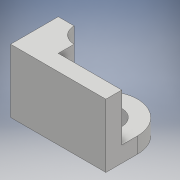
# Autodesk Inventor part: 7
Saved by Autodesk Inventor 2017 (Build 210142000, 142)
## iProperties
Part Number: 7
Material: 一般
Document SubType Name: Modeling
Designer: Brian
Density: 1 g/cm^3
Appearance: 預設
Author: Brian
Autodesk Inventor part; units mm, degrees
ref_plane "YZ Plane" through (0, 0, 0) normal (1, 0, 0) x (0, 1, 0)
ref_plane "XZ Plane" through (0, 0, 0) normal (0, 1, 0) x (-1, 0, 0)
ref_plane "XY Plane" through (0, 0, 0) normal (0, 0, 1) x (1, 0, 0)
sketch "草圖1" plane through (0, 0, 0) normal (0, 1, 0) x (-1, 0, 0)
  line L0 (0, 0) -> (-60, 0)
  line L1 (-60, 0) -> (-60, -40)
  line L2 (-60, -40) -> (0, -40)
  line L3 (0, -40) -> (0, 0)
  dimension "d0" = 60
  dimension "d1" = 40
  constraints: 8 end point, 2 parallel, 1 horizontal, 1 perpendicular
  measures "d0" distance of L0.start L0.end
  measures "d1" distance of L2.end L0.start
extrude "擠出1" add sketch "草圖1" along normal blind 10
sketch "草圖2" plane through (0, 0, 0) normal (0, 0, 1) x (1, 0, 0)
  line L0 (0, 10) -> (60, 10) projected
  line L1 (0, 10) -> (20, 10)
  line L2 (20, 10) -> (20, 30)
  line L3 (20, 30) -> (0, 30)
  line L4 (0, 30) -> (0, 10)
  point P0 (0, 0)
  dimension "d4" = 20
  dimension "d5" = 20
  constraints: 8 end point, 2 parallel, 1 horizontal, 1 perpendicular
  measures "d4" distance of L2.end L3.end
  measures "d5" distance of L3.end L0.start
extrude "擠出2" add sketch "草圖2" against normal blind 10
sketch "草圖3" plane through (60, 0, -40) normal (0, 0, -1) x (-1, 0, 0)
  line L0 (0, 10) -> (60, 10) projected
  line L1 (0, 10) -> (40, 10)
  line L2 (40, 10) -> (40, 40)
  line L3 (40, 40) -> (0, 40)
  line L4 (0, 40) -> (0, 10)
  line L5 (60, 0) -> (60, 30) projected
  line L6 (40, 10) -> (60, 10)
  line L7 (60, 10) -> (60, 20)
  line L8 (60, 20) -> (40, 20)
  line L9 (40, 20) -> (40, 10)
  dimension "d8" = 20
  dimension "d9" = 30
  dimension "d10" = 10
  constraints: 16 end point, 4 parallel, 2 horizontal, 2 perpendicular, 1 point on line
  measures "d8" distance of L7.end L8.end
  measures "d9" distance of L3.end L0.start
  measures "d10" distance between parallel lines of L0 L8
extrude "擠出3" add sketch "草圖3" against normal blind 10
fillet "圓角1" radius 20 2 edges at (60, 40, -35) (20, 40, -35)
sketch "草圖4" plane through (60, 0, -40) normal (0, 0, -1) x (-1, 0, 0)
  arc A0 (40, 20) -> (0, 20) centre (20, 20) ccw projected
  circle A1 centre (20, 20) radius 10
  point P0 (60, 0)
  dimension "d15" = 20
  constraints: 1 centre point, 1 coincident
  measures "d15" diameter of A1
extrude "擠出4" cut sketch "草圖4" against normal blind 10
sketch "草圖5" plane through (0, 0, 0) normal (0, 0, 1) x (1, 0, 0)
  circle A0 centre (20, 30) radius 10
  point P0 (0, 0)
  dimension "d18" = 20
  constraints: 1 centre point
  measures "d18" diameter of A0
extrude "擠出5" cut sketch "草圖5" against normal blind 10
